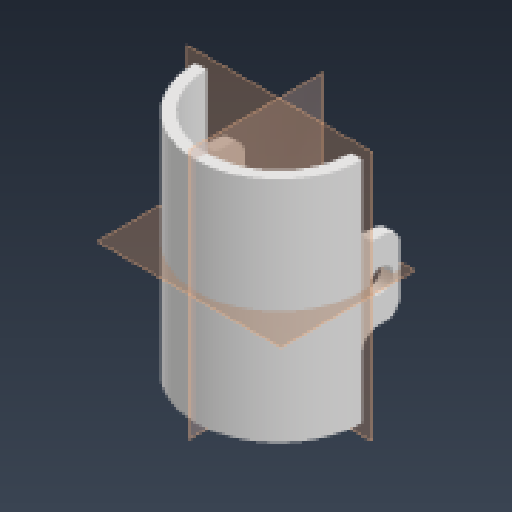
# Autodesk Inventor part: Крепление_маркера
Saved by Autodesk Inventor 2023.2 (Build 272271030, 271C)
## iProperties
Created: 2026-01-04
Part Number: Крепление_маркера
Material: Типовые
Document SubType Name: Modeling
Designer: Олег Коноваленко
Density: 1 g/cm^3
Appearance: По умолчанию
Author: Олег Коноваленко
Autodesk Inventor part; units mm, degrees
sketch "Эскиз1" plane through (0, 0, 0) normal (0, 1, 0) x (-1, 0, 0)
  circle A0 centre (0, 0) radius 4
  circle A1 centre (0, 0) radius 9.5
  circle A2 centre (0, 0) radius 11
  line L0 (11, 0) -> (-11, 0)
  point P0 (9.5, 0)
  point P1 (-9.5, 0)
  dimension "d0" = 8
  dimension "d1" = 19
  dimension "d2" = 22
  constraints: 3 centre point, 3 coincident, 2 end point, 2 point on circle, 1 horizontal, 1 midpoint
  measures "d0" diameter of A0
  measures "d1" diameter of A1
  measures "d2" diameter of A2
extrude "Выдавливание1" add sketch "Эскиз1" along normal mid plane 30 contours A1 L0 A2 picked at (-10.3014, 1.6353)
sketch "Эскиз2" plane through (0, 0, 0) normal (0, 1, 0) x (-1, 0, 0)
  line L0 (-11, 0) -> (-9.5, 0) projected
  line L1 (-9.5, 0) -> (-11, 0)
  line L2 (-11, 0) -> (-11, -5)
  line L3 (-11, -5) -> (-9.5, -5)
  line L4 (-9.5, -5) -> (-9.5, 0)
  point P0 (0, 0)
  dimension "d5" = 5
  constraints: 8 end point, 2 parallel, 1 horizontal, 1 perpendicular
  measures "d5" distance of L0.start L2.end
extrude "Выдавливание2" add sketch "Эскиз2" along normal mid plane 10
fillet "Сопряжение1" radius 2 4 edges at (10.25, -5, 0) (10.25, 5, 0) (10.25, 5, -5) (10.25, -5, -5)
mirror "Зеркальное отражение1" about plane through (0, 0, 0) normal (1, 0, 0) of "Выдавливание2", "Сопряжение1"
sketch "Эскиз3" plane through (11, -7, 0) normal (1, 0, 0) x (0, 0, -1)
  circle A0 centre (2.5, 7) radius 1.5
  line L0 (-14.2, 7) -> (8.2, 7) construction
  line L1 (5, 4) -> (5, 10) projected
  point P0 (0, 7)
  dimension "d9" = 3
  dimension "d10" = 2.5
  constraints: 1 centre point, 1 point on line
  measures "d9" diameter of A0
  measures "d10" distance from line of L1 A0.centre
extrude "Выдавливание3" cut sketch "Эскиз3" against normal up to surface (22 mm away)
fillet "Сопряжение2" radius 2 4 edges at (10.25, 15, 0) (-10.25, 15, 0) (10.25, -15, 0) (-10.25, -15, 0)
